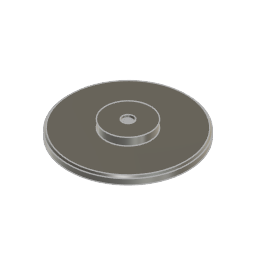
Sandblaster Window Pegs (Autodesk Fusion 360 design; units mm, degrees)
Autodesk Fusion 360 part; units mm, degrees
note: some values were not read from the file. Chosen so that the rebuilt part matches the saved one: which face or edge a step refers to; where a thread starts.
cylinder "CylinderPrimitive1" add diameter 50.8 height 3.175 placed x (1, 0, 0) y (0, 1, 0) z (0, 0, 1) at (0, 0, 0) in component "Sandblaster Cabinet pegs"
cylinder "CylinderPrimitive2" add diameter 19.05 height 3.175 placed x (1, 0, 0) y (0, 1, 0) z (0, 0, 1) at (0, 0, 3.175) in component "Sandblaster Cabinet pegs"
hole "Hole1" at (0, 0, 6.35) direction (0, 0, -1) diameter 3.429 end through all countersink diameter 4.7625 countersink angle 82 in component "Sandblaster Cabinet pegs"
thread "Thread1" "ANSI Unified Screw Threads 0.164(#8) 8-32 UNC 8-32 UNC 2B" major diameter 4.1656 minor diameter 3.4163 pitch 0.7937 angle 60 modelled right hand crest width 0.2341 on face at (0.0855, -1.7124, 3.722) crest through (0, -1.7082, 5.9799) in component "Sandblaster Cabinet pegs"
chamfer "Chamfer1" distance 0.7937 angle 45 1 edges at (-23.6811, -9.185, 3.175) in component "Sandblaster Cabinet pegs"
component "Sandblaster Cabinet pegs" placed x (1, 0, 0) y (0, 1, 0) z (0, 0, 1) at (0, 0, 0)
equation "d12 = ( 1 / 32 ) * 1 in"
